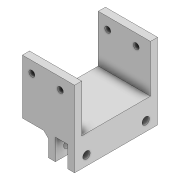
# Autodesk Inventor part: Bar_motor_mount
Saved by Autodesk Inventor 2022 (Build 260153000, 153)
## iProperties
Created: 2022-08-26
Part Number: Bar_motor_mount
Material: Generic
Document SubType Name: Modeling
Designer: dell
Density: 1 g/cm^3
Appearance: Default
Mass: 6.63054 g
Surface Area: 53.5397 cm^2
Volume: 6.63054 cm^3
Author: dell
Autodesk Inventor part; units mm, degrees
ref_plane "YZ Plane" through (0, 0, 0) normal (1, 0, 0) x (0, 1, 0)
ref_plane "XZ Plane" through (0, 0, 0) normal (0, 1, 0) x (-1, 0, 0)
ref_plane "XY Plane" through (0, 0, 0) normal (0, 0, 1) x (1, 0, 0)
sketch "Sketch1" plane through (0, 0, 0) normal (0, 1, 0) x (-1, 0, 0)
  line L0 (0, 14.5) -> (22, 14.5)
  line L1 (22, 14.5) -> (22, -14.5)
  line L2 (22, -14.5) -> (0, -14.5)
  line L3 (0, -14.5) -> (0, 14.5)
  circle A0 centre (5, 8) radius 1.25
  circle A1 centre (5, -8) radius 1.25
  circle A2 centre (17, 8) radius 1.25
  circle A3 centre (17, -8) radius 1.25
  line L4 (0, 14.5) -> (22, 14.5)
  line L5 (22, 14.5) -> (22, 17.5)
  line L6 (22, 17.5) -> (0, 17.5)
  line L7 (0, 17.5) -> (0, 14.5)
  line L8 (0, -14.5) -> (22, -14.5)
  line L9 (22, -14.5) -> (22, -17.5)
  line L10 (22, -17.5) -> (0, -17.5)
  line L11 (0, -17.5) -> (0, -14.5)
  point P0 (0, 0)
  dimension "d0" = 29
  dimension "d1" = 14.5
  dimension "d3" = 2.5
  dimension "d4" = 2.5
  dimension "d5" = 16
  dimension "d6" = 8
  dimension "d7" = 5
  dimension "d8" = 5
  dimension "d9" = 2.5
  dimension "d10" = 2.5
  dimension "d11" = 12
  dimension "d12" = 12
  dimension "d13" = 5
  dimension "d24" = 3
  dimension "d25" = 3
  constraints: 24 end point, 6 parallel, 4 centre point, 3 horizontal, 3 perpendicular, 1 midpoint
  measures "d0" distance between parallel lines of L2 L0
  measures "d1" distance from line of point (0, 0) L2
  measures "d3" diameter of A0
  measures "d4" diameter of A1
  measures "d5" distance of A0.centre A1.centre
  measures "d6" vertical distance of point (0, 0) A1.centre
  measures "d7" distance from line of L3 A0.centre
  measures "d8" distance from line of L3 A1.centre
  measures "d9" diameter of A2
  measures "d10" diameter of A3
  measures "d11" distance of A0.centre A2.centre
  measures "d12" distance of A1.centre A3.centre
  measures "d13" distance from line of L1 A2.centre
  measures "d24" distance between parallel lines of L0 L6
  measures "d25" distance between parallel lines of L2 L10
extrude "Extrusion1" add sketch "Sketch1" along normal blind 3 contours L7 L6 L5 L0 | L0 L1 L2 L3 | L2 L9 L10 L11 | A0 | A1 | A2 | A3
sketch "Sketch2" plane through (0, 0, 0) normal (0, -1, 0) x (1, 0, 0)
  line L0 (-3, 17.5) -> (0, 17.5)
  line L1 (0, 17.5) -> (0, -17.5)
  line L2 (0, -17.5) -> (-3, -17.5)
  line L3 (-3, -17.5) -> (-3, 17.5)
  line L4 (-22, 17.5) -> (0, 17.5) projected
  line L5 (0, -17.5) -> (-22, -17.5) projected
  line L6 (-22, 17.5) -> (0, 17.5) projected
  line L7 (0, -17.5) -> (-22, -17.5) projected
  line L8 (-8, 17.5) -> (-11, 17.5)
  line L9 (-11, 17.5) -> (-11, -17.5)
  line L10 (-11, -17.5) -> (-8, -17.5)
  line L11 (-8, -17.5) -> (-8, 17.5)
  line L12 (0, 17.5) -> (0, -17.5) projected
  point P0 (0, 0)
  point P1 (-8, -17.5)
  dimension "d17" = 3
  dimension "d40" = 3
  dimension "d41" = 5
  dimension "d50" = 0
  constraints: 16 end point, 4 parallel, 2 collinear, 2 horizontal, 2 perpendicular, 1 midpoint, 1 point on line
  measures "d17" distance between parallel lines of L3 L1
  measures "d40" distance between parallel lines of L9 L11
  measures "d41" distance between parallel lines of L3 L11
  measures "d50" distance between parallel lines of L12 L1
extrude "Extrusion2" add sketch "Sketch2" along normal blind 9 contours L0 L1 L2 L3 | L11 L5 L9 L4
sketch "Sketch5" plane through (0, 3, 0) normal (0, 1, 0) x (1, 0, 0)
  line L0 (-22, -17.5) -> (0, -17.5) projected
  line L1 (-22, -17.5) -> (0, -17.5)
  line L2 (0, -17.5) -> (0, -14.5)
  line L3 (0, -14.5) -> (-22, -14.5)
  line L4 (-22, -14.5) -> (-22, -17.5)
  line L5 (-22, 17.5) -> (0, 17.5)
  line L6 (0, 17.5) -> (0, 14.5)
  line L7 (0, 14.5) -> (-22, 14.5)
  line L8 (-22, 14.5) -> (-22, 17.5)
  line L9 (0, 17.5) -> (-22, 17.5) projected
  line L10 (0, -17.5) -> (0, 17.5) projected
  point P0 (0, 0)
  dimension "d26" = 3
  dimension "d27" = 3
  constraints: 16 end point, 4 parallel, 3 collinear, 2 horizontal, 2 perpendicular, 1 point on line
  measures "d26" distance between parallel lines of L0 L3
  measures "d27" distance between parallel lines of L5 L7
extrude "Extrusion4" add sketch "Sketch5" along normal blind 20
sketch "Sketch6" plane through (0, 0, 17.5) normal (0, 0, 1) x (1, 0, 0)
  circle A0 centre (-18, 18.25) radius 1.25
  line L0 (-22, 0) -> (0, 0) construction
  circle A1 centre (-6, 18.25) radius 1.25
  line L1 (-22, 0) -> (-22, 23) projected
  line L2 (0, 0) -> (0, 23) projected
  line L3 (-22, 3) -> (0, 3) projected
  line L4 (0, 3) -> (-22, 3) projected
  dimension "d34" = 2.5
  dimension "d53" = 2.5
  dimension "d54" = 4
  dimension "d55" = 6
  dimension "d56" = 15.25
  dimension "d57" = 15.25
  constraints: 2 centre point
  measures "d34" diameter of A0
  measures "d53" diameter of A1
  measures "d54" distance from line of L1 A0.centre
  measures "d55" distance from line of L2 A1.centre
  measures "d56" distance from line of L4 A0.centre
  measures "d57" distance from line of L3 A1.centre
extrude "Extrusion5" cut sketch "Sketch6" against normal blind 50
sketch "Sketch8" plane through (0, -9, 17.5) normal (1, 0, 0) x (0, 0, -1)
  circle A0 centre (5, 4) radius 1.55
  circle A1 centre (30, 4) radius 1.55
  line L0 (35, 0) -> (0, 0) projected
  line L1 (35, 0) -> (0, 0) projected
  line L2 (35, 0) -> (35, 32) projected
  line L3 (0, 0) -> (0, 32) projected
  point P0 (17.5, 9)
  dimension "d42" = 3.1
  dimension "d43" = 3.1
  dimension "d46" = 4
  dimension "d47" = 4
  dimension "d65" = 5
  dimension "d66" = 5
  constraints: 2 centre point
  measures "d42" diameter of A0
  measures "d43" diameter of A1
  measures "d46" distance from line of L0 A0.centre
  measures "d47" distance from line of L1 A1.centre
  measures "d65" distance from line of L2 A1.centre
  measures "d66" distance from line of L3 A0.centre
extrude "Extrusion6" cut sketch "Sketch8" against normal blind 100
thicken "Thicken1" operation add thickness 0.1 both sides no extend neighbours yes toward (1, 0, 0) faces at (-3, -1.1836, -3.9835)
thicken "Thicken2" operation add thickness 0.1 both sides no extend neighbours yes toward (-1, 0, 0) faces at (-8, -1.1836, -3.9835)
chamfer "Chamfer1" distance 2 angle 45 1 edges at (-11, 0, 0)
equation "\"d1\" = 0.5 * d0"
equation "\"d6\" = 0.5 * d5"
body "Solid1"
